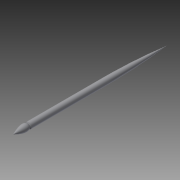
# Autodesk Inventor part: brush
Saved by Autodesk Inventor 2013 (Build 170138000, 138)
## iProperties
Created: 2017-01-26
Part Number: brush
Material: Generic
Document SubType Name: Modeling
Designer: Herman de Vries
Density: 1 g/cm^3
Author: Herman de Vries
Autodesk Inventor part; units mm, degrees
ref_plane "YZ Plane" through (0, 0, 0) normal (1, 0, 0) x (0, 1, 0)
ref_plane "XZ Plane" through (0, 0, 0) normal (0, 1, 0) x (-1, 0, 0)
ref_plane "XY Plane" through (0, 0, 0) normal (0, 0, 1) x (1, 0, 0)
sketch "Sketch1" plane through (0, 0, 0) normal (0, 0, 1) x (1, 0, 0)
  line L0 (0, 0) -> (0, 200)
  arc A0 (4, 120) -> (0, 200) centre (-798, 120) ccw
  line L1 (4, 120) -> (4, 20)
  spline S0 degree 2 poles (0, 0) (7.0841, 14.8032) (2.7488, 19.0626) knots 0 0 0 1 1 1
  line L2 (4, 20) -> (2.7488, 19.0626)
  point P0 (4.3878, 14.7086)
  dimension "d1" = 200
  dimension "d2" = 8
  dimension "d3" = 100
  dimension "d4" = 20
  constraints: 6 end point, 2 point on circle, 1 centre point, 1 parallel, 1 tangent, 1 vertical, 3 other
  measures "d1" distance of L0.start L0.end
  measures "d2" diameter of L1 L0
  measures "d3" distance of L1.start L1.end
  measures "d4" vertical distance of L1.end L0.start
revolve "Revolution1" add sketch "Sketch1" angle 360 about axis through (0, 0, 0) along (0, 1, 0)
body "Solid1"
